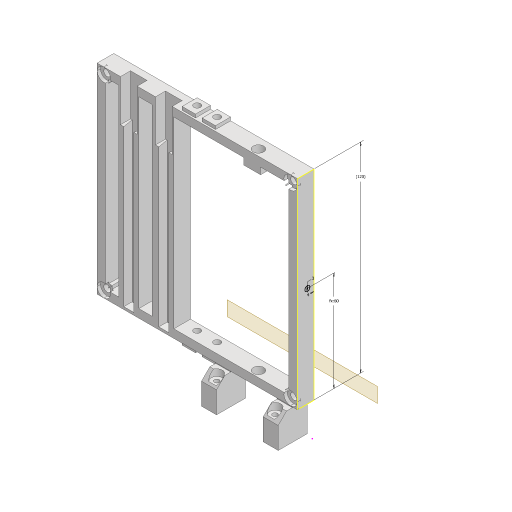
# Autodesk Inventor part: Rail_stage_x_m6_v2
Saved by Autodesk Inventor 2023 (Build 270158000, 158)
## iProperties
Created: 2020-12-08
Part Number: Rail_stage_x_m6_v2
Material: Generic
Document SubType Name: Modeling
Designer: CDT
Density: 1 g/cm^3
Appearance: Default
Author: CDT
Autodesk Inventor part; units mm, degrees
ref_plane "YZ Plane" through (0, 0, 0) normal (1, 0, 0) x (0, 1, 0)
ref_plane "XZ Plane" through (0, 0, 0) normal (0, 1, 0) x (-1, 0, 0)
ref_plane "XY Plane" through (0, 0, 0) normal (0, 0, 1) x (1, 0, 0)
ref_plane "Work Plane1" through (34.0618, 17.7005, 0) normal (0, 0, 1) x (1, 0, 0)
sketch "Sketch1" plane through (34.0618, 17.7005, 0) normal (0, 0, 1) x (1, 0, 0)
  line L0 (-34.0618, -17.7005) -> (-154.0618, -17.7005)
  line L1 (-154.0618, -17.7005) -> (-154.0618, 102.2995)
  line L2 (-154.0618, 102.2995) -> (-34.0618, 102.2995)
  line L3 (-34.0618, 102.2995) -> (-34.0618, -17.7005)
  circle A0 centre (-38.0618, 98.2995) radius 2
  circle A1 centre (-38.0618, -13.7005) radius 2
  circle A2 centre (-150.0618, -13.7005) radius 2
  circle A3 centre (-150.0618, 98.2995) radius 2
  dimension "d0" = 120
  dimension "d1" = 120
  dimension "d2" = 4
  dimension "d3" = 4
  dimension "d4" = 4
  dimension "d5" = 4
  dimension "d6" = 4
  dimension "d7" = 4
  dimension "d8" = 4
  dimension "d9" = 4
  dimension "d10" = 4
  dimension "d11" = 4
  dimension "d12" = 4
  dimension "d13" = 4
  constraints: 8 end point, 4 centre point, 2 parallel, 1 horizontal, 1 perpendicular
  measures "d0" distance of L1.end L2.end
  measures "d1" distance of L0.end L1.end
  measures "d2" diameter of A0
  measures "d3" diameter of A1
  measures "d4" diameter of A2
  measures "d5" diameter of A3
  measures "d6" distance from line of L2 A3.centre
  measures "d7" distance from line of L1 A3.centre
  measures "d8" distance from line of L1 A2.centre
  measures "d9" distance from line of L0 A2.centre
  measures "d10" distance from line of L3 A1.centre
  measures "d11" distance from line of L0 A1.centre
  measures "d12" distance from line of L3 A0.centre
  measures "d13" distance from line of L2 A0.centre
extrude "Extrusion1" add sketch "Sketch1" along normal blind 10
sketch "Sketch44" plane through (34.0618, 17.7005, 0) normal (0, 0, -1) x (-1, 0, 0)
  line L0 (84.0618, -17.7005) -> (75.0618, -17.7005)
  line L1 (75.0618, -17.7005) -> (75.0618, -37.2005)
  line L2 (75.0618, -37.2005) -> (84.0618, -37.2005)
  line L3 (84.0618, -37.2005) -> (84.0618, -17.7005)
  line L4 (154.0618, -17.7005) -> (34.0618, -17.7005) projected
  line L5 (47.0618, -17.7005) -> (38.0618, -17.7005)
  line L6 (38.0618, -17.7005) -> (38.0618, -37.2005)
  line L7 (38.0618, -37.2005) -> (47.0618, -37.2005)
  line L8 (47.0618, -37.2005) -> (47.0618, -17.7005)
  line L9 (154.0618, 102.2995) -> (154.0618, -17.7005) projected
  line L10 (34.0618, -17.7005) -> (34.0618, 102.2995) projected
  point P0 (96.0618, -9.1005)
  point P1 (102.0618, -9.1005)
  dimension "d454" = 9
  dimension "d455" = 19.5
  dimension "d456" = 9
  dimension "d457" = 19.5
  dimension "d1352" = 4
  dimension "d1353" = 28
  constraints: 16 end point, 4 parallel, 2 horizontal, 2 perpendicular, 1 collinear, 1 point on line
  measures "d454" distance of L2.end L1.end
  measures "d455" distance of L1.end L0.end
  measures "d456" distance of L7.end L6.end
  measures "d457" distance of L6.end L5.end
  measures "d1352" distance between parallel lines of L10 L6
  measures "d1353" distance between parallel lines of L1 L8
extrude "Extrusion41" add sketch "Sketch44" against normal blind 8.9
sketch "Sketch67" plane through (34.0618, 17.7005, 0) normal (0, 0, -1) x (-1, 0, 0)
  line L0 (92.0618, -17.7005) -> (84.0618, -17.7005)
  line L1 (84.0618, -17.7005) -> (84.0618, -19.7005)
  line L2 (84.0618, -19.7005) -> (92.0618, -19.7005)
  line L3 (92.0618, -19.7005) -> (92.0618, -17.7005)
  line L4 (96.0618, -17.7005) -> (104.0618, -17.7005)
  line L5 (104.0618, -17.7005) -> (104.0618, -19.7005)
  line L6 (104.0618, -19.7005) -> (96.0618, -19.7005)
  line L7 (96.0618, -19.7005) -> (96.0618, -17.7005)
  line L8 (84.0618, -37.2005) -> (84.0618, -17.7005) projected
  line L9 (154.0618, -17.7005) -> (84.0618, -17.7005) projected
  line L10 (154.0618, -17.7005) -> (34.0618, -17.7005) projected
  line L11 (104.0618, 104.2995) -> (96.0618, 104.2995)
  line L12 (96.0618, 104.2995) -> (96.0618, 102.2995)
  line L13 (96.0618, 102.2995) -> (104.0618, 102.2995)
  line L14 (104.0618, 102.2995) -> (104.0618, 104.2995)
  line L15 (92.0618, 104.2995) -> (84.0618, 104.2995)
  line L16 (84.0618, 104.2995) -> (84.0618, 102.2995)
  line L17 (84.0618, 102.2995) -> (92.0618, 102.2995)
  line L18 (92.0618, 102.2995) -> (92.0618, 104.2995)
  line L19 (34.0618, 102.2995) -> (154.0618, 102.2995) projected
  line L20 (154.0618, 102.2995) -> (154.0618, -17.7005) projected
  line L21 (34.0618, -17.7005) -> (34.0618, 102.2995) projected
  point P0 (116.5618, -23.7005)
  point P1 (122.5618, -17.7005)
  point P2 (65.5618, -17.7005)
  dimension "d861" = 8
  dimension "d862" = 2
  dimension "d863" = 8
  dimension "d864" = 2
  dimension "d866" = 0
  dimension "d868" = 0
  dimension "d869" = 8
  dimension "d870" = 2
  dimension "d871" = 8
  dimension "d872" = 2
  dimension "d1350" = 50
  dimension "d1351" = 50
  constraints: 32 end point, 8 parallel, 4 collinear, 4 horizontal, 4 perpendicular, 1 other
  measures "d861" distance of L2.end L1.end
  measures "d862" distance of L1.end L0.end
  measures "d863" distance of L5.end L6.end
  measures "d864" distance of L4.end L5.end
  measures "d866" distance between parallel lines of L9 L4
  measures "d868" distance between parallel lines of L10 L0
  measures "d869" distance between parallel lines of L12 L14
  measures "d870" distance between parallel lines of L19 L11
  measures "d871" distance between parallel lines of L16 L18
  measures "d872" distance between parallel lines of L19 L15
  measures "d1350" distance between parallel lines of L20 L5
  measures "d1351" distance between parallel lines of L21 L1
extrude "Extrusion61" add sketch "Sketch67" against normal blind 9 contours L3 L2 L1 L0 | L4 L5 L6 L7 | L16 L15 L18 L17 | L13 L12 L11 L14
sketch "Sketch68" plane through (-58, -2, 0) normal (0, -1, 0) x (1, 0, 0)
  circle A0 centre (4, 4) radius 2
  line L0 (8, 8.9) -> (8, 9) projected
  line L1 (0, 9) -> (8, 9) projected
  circle A1 centre (-8, 4) radius 2
  line L2 (-12, 9) -> (-4, 9) projected
  line L3 (-4, 0) -> (-4, 9) projected
  line L4 (-4, 0) -> (-12, 0) projected
  point P0 (58, 0)
  point P1 (8, 0)
  point P2 (-53, 8.8)
  dimension "d875" = 4
  dimension "d876" = 4
  dimension "d877" = 5
  dimension "d878" = 4
  dimension "d879" = 5
  dimension "d880" = 4
  dimension "d1039" = 4
  constraints: 2 centre point, 1 other
  measures "d875" diameter of A0
  measures "d876" distance from line of L0 A0.centre
  measures "d877" distance from line of L1 A0.centre
  measures "d878" diameter of A1
  measures "d879" distance from line of L2 A1.centre
  measures "d1039" distance from line of L4 A1.centre
extrude "Extrusion62" cut sketch "Sketch68" against normal blind 7
sketch "Sketch69" plane through (-70, 122, 0) normal (0, 1, 0) x (1, 0, 0)
  circle A0 centre (4, -4) radius 2 projected
  circle A1 centre (4, -4) radius 2
  line L0 (12, 0) -> (20, 0) projected
  line L1 (0, 0) -> (8, 0) projected
  circle A2 centre (16, -4) radius 2 projected
  circle A3 centre (16, -4) radius 2
  dimension "d1038" = 4
  constraints: 2 centre point, 2 coincident
  measures "d1038" distance from line of L1 A1.centre
extrude "Extrusion63" cut sketch "Sketch69" against normal blind 7
chamfer "Chamfer54" distance 1.5 angle 45 1 edges at (-13, 0, 4.45)
sketch "Sketch106" plane through (0, 0, 10) normal (1, 0, 0) x (0, 0, -1)
  circle A0 centre (6, 60) radius 1.5
  line L0 (0, 0) -> (0, 120) projected
  line L1 (10, 120) -> (0, 120) projected
  line L2 (1.1, 0) -> (10, 0) projected
  line L3 (10, 0) -> (10, 120) projected
  point P0 (9, -19.5)
  dimension "d1499" = 3
  dimension "d1501" = 120
  dimension "d1502" = 60
  dimension "d1505" = 4
  constraints: 1 centre point, 1 other
  measures "d1499" diameter of A0
  measures "d1501" distance between parallel lines of L1 L2
  measures "d1502" distance from line of A0.centre L2
sketch "Sketch108" plane through (-120, 0, 0) normal (-1, 0, 0) x (0, 0, 1)
  circle A0 centre (4.1, 60) radius 1.5
  line L0 (0, 120) -> (0, 0) projected
  line L1 (0, 120) -> (10, 120) projected
  line L2 (0, 0) -> (10, 0) projected
  dimension "d1513" = 3
  dimension "d1514" = 4.1
  dimension "d1515" = 60
  dimension "d1516" = 120
  constraints: 1 centre point
  measures "d1513" diameter of A0
  measures "d1514" distance from line of L0 A0.centre
  measures "d1515" distance from line of L1 A0.centre
  measures "d1516" distance between parallel lines of L2 L1
extrude "Extrusion98" cut sketch "Sketch108" against normal blind 3.5
sketch "Sketch110" plane through (34.0618, 17.7005, 10) normal (0, 0, 1) x (1, 0, 0)
  line L0 (-149.0618, 97.2995) -> (-39.0618, 97.2995)
  line L1 (-39.0618, 97.2995) -> (-39.0618, -12.7005)
  line L2 (-39.0618, -12.7005) -> (-149.0618, -12.7005)
  line L3 (-149.0618, -12.7005) -> (-149.0618, 97.2995)
  line L4 (-154.0618, 102.2995) -> (-154.0618, -17.7005) projected
  line L5 (-34.0618, 102.2995) -> (-154.0618, 102.2995) projected
  line L6 (-34.0618, -17.7005) -> (-34.0618, 102.2995) projected
  line L7 (-154.0618, -17.7005) -> (-34.0618, -17.7005) projected
  line L8 (-34.0618, -17.7005) -> (-41.0618, -17.7005)
  line L9 (-41.0618, -17.7005) -> (-41.0618, -10.7005)
  line L10 (-41.0618, -10.7005) -> (-34.0618, -10.7005)
  line L11 (-34.0618, -10.7005) -> (-34.0618, -17.7005)
  line L12 (-154.0618, -17.7005) -> (-34.0618, -17.7005) projected
  line L13 (-154.0618, -17.7005) -> (-147.0618, -17.7005)
  line L14 (-147.0618, -17.7005) -> (-147.0618, -10.7005)
  line L15 (-147.0618, -10.7005) -> (-154.0618, -10.7005)
  line L16 (-154.0618, -10.7005) -> (-154.0618, -17.7005)
  line L17 (-154.0618, 102.2995) -> (-147.0618, 102.2995)
  line L18 (-147.0618, 102.2995) -> (-147.0618, 95.2995)
  line L19 (-147.0618, 95.2995) -> (-154.0618, 95.2995)
  line L20 (-154.0618, 95.2995) -> (-154.0618, 102.2995)
  line L21 (-34.0618, 102.2995) -> (-154.0618, 102.2995) projected
  line L22 (-34.0618, 102.2995) -> (-41.0618, 102.2995)
  line L23 (-41.0618, 102.2995) -> (-41.0618, 95.2995)
  line L24 (-41.0618, 95.2995) -> (-34.0618, 95.2995)
  line L25 (-34.0618, 95.2995) -> (-34.0618, 102.2995)
  line L26 (-66.0618, 93.2995) -> (-56.0618, 93.2995)
  line L27 (-56.0618, 93.2995) -> (-56.0618, 97.2995)
  line L28 (-56.0618, 97.2995) -> (-66.0618, 97.2995)
  line L29 (-66.0618, 97.2995) -> (-66.0618, 93.2995)
  point P0 (-104.0618, 102.2995)
  point P1 (-84.0618, -17.7005)
  point P2 (-104.0618, -17.7005)
  point P3 (-84.0618, 102.2995)
  point P4 (-39.0618, 95.2995)
  point P5 (-41.0618, 97.2995)
  point P6 (-147.0618, 97.2995)
  point P7 (-149.0618, 95.2995)
  point P8 (-149.0618, -10.7005)
  point P9 (-147.0618, -12.7005)
  point P10 (-41.0618, -12.7005)
  point P11 (-39.0618, -10.7005)
  dimension "d1532" = 5
  dimension "d1533" = 5
  dimension "d1534" = 5
  dimension "d1535" = 5
  dimension "d1609" = 7
  dimension "d1610" = 7
  dimension "d1611" = 7
  dimension "d1612" = 7
  dimension "d1613" = 7
  dimension "d1614" = 7
  dimension "d1615" = 7
  dimension "d1616" = 7
  dimension "d1640" = 17
  dimension "d1641" = 10
  dimension "d1642" = 4
  constraints: 48 end point, 12 parallel, 6 horizontal, 6 perpendicular, 1 point on line
  measures "d1532" distance between parallel lines of L4 L3
  measures "d1533" distance between parallel lines of L5 L0
  measures "d1534" distance between parallel lines of L6 L1
  measures "d1535" distance between parallel lines of L7 L2
  measures "d1609" distance of L9.end L10.end
  measures "d1610" distance of L8.end L9.end
  measures "d1611" distance of L15.end L14.end
  measures "d1612" distance of L14.end L13.end
  measures "d1613" distance of L18.end L19.end
  measures "d1614" distance of L17.end L18.end
  measures "d1615" distance of L24.end L23.end
  measures "d1616" distance of L23.end L22.end
  measures "d1640" distance between parallel lines of L27 L1
  measures "d1641" distance between parallel lines of L29 L27
  measures "d1642" distance between parallel lines of L28 L26
extrude "Extrusion100" cut sketch "Sketch110" against normal through all contours L29 L26 L27 L0 L23 L24 L1 L10 L9 L2 L14 L15 L3 L19 L18
sketch "Sketch115" plane through (34.0618, 17.7005, 0) normal (0, 0, -1) x (-1, 0, 0)
  line L0 (108.0618, 102.2995) -> (121.0618, 102.2995)
  line L1 (121.0618, 102.2995) -> (121.0618, -17.7005)
  line L2 (121.0618, -17.7005) -> (108.0618, -17.7005)
  line L3 (108.0618, -17.7005) -> (108.0618, 102.2995)
  line L4 (129.0618, 102.2995) -> (141.0618, 102.2995)
  line L5 (141.0618, 102.2995) -> (141.0618, -17.7005)
  line L6 (141.0618, -17.7005) -> (129.0618, -17.7005)
  line L7 (129.0618, -17.7005) -> (129.0618, 102.2995)
  line L8 (34.0618, -17.7005) -> (34.0618, 102.2995) projected
  line L9 (149.0618, 95.2995) -> (149.0618, -10.7005) projected
  line L10 (104.0618, 102.2995) -> (154.0618, 102.2995) projected
  line L11 (154.0618, -17.7005) -> (104.0618, -17.7005) projected
  line L12 (75.0618, -17.7005) -> (48.5618, -17.7005) projected
  line L13 (34.0618, 102.2995) -> (84.0618, 102.2995) projected
  line L14 (154.0618, 102.2995) -> (154.0618, -17.7005) projected
  point P0 (149.0618, 96.5674)
  point P1 (149.0618, -11.9685)
  dimension "d1577" = 13
  dimension "d1578" = 8
  dimension "d1579" = 12
  dimension "d1580" = 0
  dimension "d1581" = 0
  dimension "d1582" = 0
  dimension "d1583" = 0
  dimension "d1598" = 33
  constraints: 16 end point, 4 parallel, 2 horizontal, 2 perpendicular
  measures "d1577" distance between parallel lines of L1 L3
  measures "d1578" distance between parallel lines of L9 L5
  measures "d1579" distance between parallel lines of L7 L5
  measures "d1580" distance between parallel lines of L10 L4
  measures "d1581" distance between parallel lines of L11 L6
  measures "d1582" distance between parallel lines of L12 L2
  measures "d1583" distance between parallel lines of L13 L0
  measures "d1598" distance between parallel lines of L14 L1
extrude "Extrusion104" add sketch "Sketch115" against normal up to surface (10 mm away) contours L0 L1 L2 L3 | L4 L5 L6 L7
sketch "Sketch116" plane through (34.0618, 17.7005, 10) normal (0, 0, 1) x (1, 0, 0)
  line L0 (-111.0618, -16.2005) -> (-117.0618, -16.2005)
  line L1 (-117.0618, -16.2005) -> (-117.0618, 102.2995)
  line L2 (-117.0618, 102.2995) -> (-111.0618, 102.2995)
  line L3 (-111.0618, 102.2995) -> (-111.0618, -16.2005)
  line L4 (-132.0618, -16.2005) -> (-138.0618, -16.2005)
  line L5 (-138.0618, -16.2005) -> (-138.0618, 102.2995)
  line L6 (-138.0618, 102.2995) -> (-132.0618, 102.2995)
  line L7 (-132.0618, 102.2995) -> (-132.0618, -16.2005)
  line L8 (-154.0618, -17.7005) -> (-34.0618, -17.7005) projected
  line L9 (-34.0618, 102.2995) -> (-154.0618, 102.2995) projected
  line L10 (-34.0618, -17.7005) -> (-34.0618, 102.2995) projected
  line L11 (-108.0618, 97.2995) -> (-108.0618, -12.7005) projected
  line L12 (-121.0618, -12.7005) -> (-108.0618, -12.7005) projected
  line L13 (-34.0618, 102.2995) -> (-154.0618, 102.2995) projected
  line L14 (-129.0618, 97.2995) -> (-129.0618, -12.7005) projected
  line L15 (-141.0618, -12.7005) -> (-129.0618, -12.7005) projected
  point P0 (-104.0618, -17.7005)
  point P1 (-84.0618, 102.2995)
  point P2 (-39.7938, -12.7005)
  point P3 (-104.0618, 102.2995)
  point P4 (-148.3297, -12.7005)
  dimension "d1587" = 0
  dimension "d1588" = 6
  dimension "d1590" = 3
  dimension "d1592" = 0
  dimension "d1593" = 3
  dimension "d1594" = 6
  dimension "d1669" = 1.5
  dimension "d1670" = 1.5
  constraints: 16 end point, 4 parallel, 2 horizontal, 2 perpendicular
  measures "d1587" distance between parallel lines of L9 L2
  measures "d1588" distance between parallel lines of L1 L3
  measures "d1590" distance between parallel lines of L11 L3
  measures "d1592" distance between parallel lines of L13 L6
  measures "d1593" distance between parallel lines of L14 L7
  measures "d1594" distance between parallel lines of L5 L7
  measures "d1669" distance between parallel lines of L8 L0
  measures "d1670" distance between parallel lines of L8 L4
extrude "Extrusion105" cut sketch "Sketch116" against normal blind 6 draft 10
sketch "Sketch117" plane through (34.0618, 17.7005, 10) normal (0, 0, 1) x (1, 0, 0)
  line L0 (-109.0618, 77.2995) -> (-119.0618, 77.2995)
  line L1 (-119.0618, 77.2995) -> (-119.0618, 102.2995)
  line L2 (-119.0618, 102.2995) -> (-109.0618, 102.2995)
  line L3 (-109.0618, 102.2995) -> (-109.0618, 77.2995)
  line L4 (-130.0618, 77.2995) -> (-140.0618, 77.2995)
  line L5 (-140.0618, 77.2995) -> (-140.0618, 102.2995)
  line L6 (-140.0618, 102.2995) -> (-130.0618, 102.2995)
  line L7 (-130.0618, 102.2995) -> (-130.0618, 77.2995)
  line L8 (-118.1197, 102.2995) -> (-110.0038, 102.2995) projected
  line L9 (-108.0618, 97.2995) -> (-108.0618, -12.7005) projected
  line L10 (-139.1197, 102.2995) -> (-131.0038, 102.2995) projected
  line L11 (-129.0618, 97.2995) -> (-129.0618, -12.7005) projected
  point P0 (-34.0618, -17.7005)
  dimension "d1599" = 10
  dimension "d1600" = 10
  dimension "d1601" = 25
  dimension "d1602" = 0
  dimension "d1603" = 1
  dimension "d1604" = 0
  dimension "d1605" = 25
  dimension "d1606" = 1
  constraints: 16 end point, 4 parallel, 2 horizontal, 2 perpendicular
  measures "d1599" distance of L5.end L6.end
  measures "d1600" distance of L1.end L2.end
  measures "d1601" distance between parallel lines of L0 L2
  measures "d1602" distance between parallel lines of L8 L2
  measures "d1603" distance between parallel lines of L9 L3
  measures "d1604" distance between parallel lines of L10 L6
  measures "d1605" distance between parallel lines of L4 L6
  measures "d1606" distance between parallel lines of L11 L7
extrude "Extrusion106" cut sketch "Sketch117" against normal up to surface (6 mm away)
sketch "Sketch118" plane through (34.0618, 17.7005, 10) normal (0, 0, 1) x (1, 0, 0)
  circle A0 centre (-38.0618, -13.7005) radius 2 projected
  circle A1 centre (-38.0618, -13.7005) radius 4
  circle A2 centre (-150.0618, -13.7005) radius 2 projected
  circle A3 centre (-150.0618, -13.7005) radius 4
  circle A4 centre (-150.0618, 98.2995) radius 2 projected
  circle A5 centre (-150.0618, 98.2995) radius 4
  circle A6 centre (-38.0618, 98.2995) radius 2 projected
  circle A7 centre (-38.0618, 98.2995) radius 4
  point P0 (-34.0618, -17.7005)
  dimension "d1617" = 8
  dimension "d1618" = 8
  dimension "d1619" = 8
  dimension "d1620" = 8
  constraints: 4 centre point, 4 coincident
  measures "d1617" diameter of A1
  measures "d1618" diameter of A3
  measures "d1619" diameter of A5
  measures "d1620" diameter of A7
extrude "Extrusion107" cut sketch "Sketch118" against normal blind 2 contours A1 | A3 | A4 | A5 | A6 | A7
sketch "Sketch119" plane through (-41, 0, 0) normal (0, -1, 0) x (1, 0, 0)
  circle A0 centre (14, 6.25) radius 3.15
  line L0 (-9, 0) -> (-9, 8.9) projected
  line L1 (37, 0) -> (37, 8.9) projected
  line L2 (0, 0) -> (26.5, 0) projected
  line L3 (-9, 9) -> (-17, 9) projected
  line L4 (-75, 10) -> (37, 10) projected
  point P0 (41, 0)
  point P1 (34, 9)
  dimension "d1623" = 6.3
  dimension "d1624" = 23
  dimension "d1625" = 23
  dimension "d1672" = 3.75
  constraints: 1 centre point
  measures "d1623" diameter of A0
  measures "d1624" distance from line of L0 A0.centre
  measures "d1625" distance from line of L1 A0.centre
  measures "d1672" distance from line of L4 A0.centre
extrude "Extrusion108" cut sketch "Sketch119" against normal through all
sketch "Sketch120" plane through (34.0618, 17.7005, 8.9) normal (0, 0, 1) x (1, 0, 0)
  line L0 (-47.0618, -37.2005) -> (-38.0618, -37.2005) projected
  line L1 (-47.0618, -19.2005) -> (-47.0618, -37.2005) projected
  line L2 (-38.0618, -37.2005) -> (-47.0618, -37.2005)
  line L3 (-47.0618, -37.2005) -> (-47.0618, -19.2005)
  line L4 (-47.0618, -19.2005) -> (-38.0618, -19.2005)
  line L5 (-38.0618, -19.2005) -> (-38.0618, -37.2005)
  line L6 (-92.0618, -19.7005) -> (-84.0618, -19.7005) projected
  line L7 (-84.0618, -37.2005) -> (-75.0618, -37.2005)
  line L8 (-75.0618, -37.2005) -> (-75.0618, -19.2005)
  line L9 (-75.0618, -19.2005) -> (-84.0618, -19.2005)
  line L10 (-84.0618, -19.2005) -> (-84.0618, -37.2005)
  line L11 (-75.0618, -37.2005) -> (-75.0618, -17.7005) projected
  line L12 (-84.0618, -17.7005) -> (-38.0618, -17.7005) projected
  point P0 (-34.0618, -17.7005)
  dimension "d1655" = 0
  dimension "d1656" = 1.5
  constraints: 16 end point, 4 parallel, 2 horizontal, 2 perpendicular
  measures "d1655" distance between parallel lines of L11 L8
  measures "d1656" distance between parallel lines of L12 L9
extrude "Extrusion109" add sketch "Sketch120" along normal blind 8.5
sketch "Sketch121" plane through (-13, -19.5, 0) normal (0, -1, 0) x (1, 0, 0)
  circle A0 centre (-31.5, 13.75) radius 1.5
  circle A1 centre (3.5, 13.75) radius 1.5
  circle A2 centre (-14, 6.25) radius 3.15 projected
  point P0 (13, 0)
  dimension "d1632" = 3
  dimension "d1633" = 3
  dimension "d1634" = 17.5
  dimension "d1635" = 17.5
  dimension "d1636" = 7.5
  dimension "d1637" = 7.5
  constraints: 2 centre point
  measures "d1632" diameter of A0
  measures "d1633" diameter of A1
  measures "d1634" horizontal distance of A1.centre A2.centre
  measures "d1635" horizontal distance of A2.centre A0.centre
  measures "d1636" vertical distance of A2.centre A1.centre
  measures "d1637" vertical distance of A0.centre A2.centre
extrude "Extrusion110" cut sketch "Sketch121" against normal through all contours A0 | A1
sketch "Sketch123" plane through (-13, -1.5, 8.9) normal (0, 1, 0) x (1, 0, 0)
  circle A0 centre (3.5, -4.85) radius 1.5 projected
  circle A1 centre (3.5, -4.85) radius 3.4
  circle A2 centre (-31.5, -4.85) radius 1.5 projected
  circle A3 centre (-31.5, -4.85) radius 3.4
  point P0 (13, 8.9)
  dimension "d1660" = 6.8
  dimension "d1661" = 6.8
  constraints: 2 centre point, 2 coincident
  measures "d1660" diameter of A1
  measures "d1661" diameter of A3
extrude "Extrusion112" cut sketch "Sketch123" against normal blind 4
chamfer "Chamfer56" distance 5 angle 45 2 edges at (-8.5, -1.5, 17.4) (-45.5, -1.5, 17.4)
body "Solid1"
